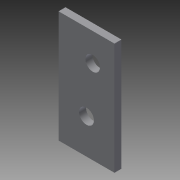
# Autodesk Inventor part: winch mount back support
Saved by Autodesk Inventor 2013 (Build 170138000, 138)
## iProperties
Created: 2013-02-09
Part Number: winch mount back support
Material: Generic
Document SubType Name: Modeling
Designer: Arpan
Density: 1 g/cm^3
Author: Arpan
Autodesk Inventor part; units mm, degrees
ref_plane "YZ Plane" through (0, 0, 0) normal (1, 0, 0) x (0, 1, 0)
ref_plane "XZ Plane" through (0, 0, 0) normal (0, 1, 0) x (-1, 0, 0)
ref_plane "XY Plane" through (0, 0, 0) normal (0, 0, 1) x (1, 0, 0)
sketch "Sketch1" plane through (0, 0, 0) normal (0, 0, 1) x (1, 0, 0)
  line L0 (0, 0) -> (-6.8345, 0)
  line L1 (-6.8345, 0) -> (18.5655, 0)
  line L2 (18.5655, 0) -> (18.5655, 50.8)
  line L3 (18.5655, 50.8) -> (-6.8345, 50.8)
  line L4 (-6.8345, 50.8) -> (-6.8345, 0)
  dimension "d0" = 25.4
  dimension "d1" = 50.8
  constraints: 10 end point, 3 perpendicular, 1 collinear, 1 horizontal
  measures "d0" distance of L0.end L1.end
  measures "d1" distance of L1.end L2.end
extrude "Extrusion1" add sketch "Sketch1" along normal blind 3.175
sketch "Sketch2" plane through (0, 0, 3.175) normal (0, 0, 1) x (1, 0, 0)
  circle A0 centre (5.8655, 15.875) radius 3.3782 projected
  circle A1 centre (8.6877, 38.1) radius 3.302 projected
  point P0 (0, 0)
extrude "Extrusion2" cut sketch "Sketch2" against normal blind 25.4
sketch "Sketch3" plane through (0, 0, 3.175) normal (0, 0, 1) x (1, 0, 0)
  line L0 (-6.8345, 0) -> (18.5655, 0) projected
  line L1 (18.5655, 0) -> (18.5655, 50.8) projected
  line L2 (-6.8345, 50.8) -> (-6.8345, 0) projected
  line L3 (-6.8345, 0) -> (-6.8345, 6.35)
  line L4 (-6.8345, 6.35) -> (18.5655, 6.35)
  point P0 (0, 0)
  dimension "d6" = 6.35
  constraints: 4 end point, 2 point on line, 1 perpendicular
  measures "d6" distance of L0.start L3.end
extrude "Extrusion3" cut sketch "Sketch3" against normal blind 25.4
body "Solid1"
